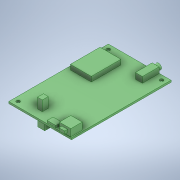
# Autodesk Inventor part: ECG PCB
Saved by Autodesk Inventor 2020 (Build 240168000, 168)
## iProperties
Created: 2021-04-18
Part Number: ECG PCB
Material: Generic
Document SubType Name: Modeling
Designer: Karl
Density: 1 g/cm^3
Appearance: Smooth - Dark Forest Green
Author: Karl
Autodesk Inventor part; units mm, degrees
ref_plane "YZ Plane" through (0, 0, 0) normal (1, 0, 0) x (0, 1, 0)
ref_plane "XZ Plane" through (0, 0, 0) normal (0, 1, 0) x (-1, 0, 0)
ref_plane "XY Plane" through (0, 0, 0) normal (0, 0, 1) x (1, 0, 0)
sketch "Sketch1" plane through (0, 0, 0) normal (0, 1, 0) x (-1, 0, 0)
  line L0 (-26.9875, 42.8625) -> (26.9875, 42.8625)
  line L1 (26.9875, 42.8625) -> (26.9875, -42.8625)
  line L2 (26.9875, -42.8625) -> (-26.9875, -42.8625)
  line L3 (-26.9875, -42.8625) -> (-26.9875, 42.8625)
  line L4 (-26.9875, 42.8625) -> (26.9875, -42.8625) construction
  line L5 (26.9875, 42.8625) -> (-26.9875, -42.8625) construction
  point P0 (0, 0)
  dimension "d0" = 53.975
  dimension "d1" = 85.725
  constraints: 12 end point, 2 midpoint, 2 parallel, 1 horizontal, 1 perpendicular
  measures "d0" distance of L1.end L2.end
  measures "d1" distance of L0.end L1.end
extrude "Extrusion1" add sketch "Sketch1" along normal blind 1.57
sketch "Sketch2" plane through (0, 1.57, 0) normal (0, 1, 0) x (1, 0, 0)
  line L0 (-26.9875, -42.8625) -> (26.9875, -42.8625) projected
  line L1 (-26.9875, 42.8625) -> (-26.9875, -42.8625) projected
  line L2 (26.9875, 42.8625) -> (-26.9875, 42.8625) projected
  line L3 (26.9875, -42.8625) -> (26.9875, 42.8625) projected
  point P0 (0, 0)
  point P1 (-22.9235, -38.7985)
  point P2 (-22.9235, 38.7985)
  point P3 (22.9235, 38.7985)
  dimension "d4" = 4.064
  dimension "d5" = 4.064
  dimension "d6" = 4.064
  dimension "d7" = 4.064
  dimension "d8" = 4.064
  dimension "d9" = 4.064
  measures "d4" distance from line of L0 point (-22.923, -38.798)
  measures "d5" distance from line of L1 point (-22.923, -38.798)
  measures "d6" distance from line of L1 point (-22.923, 38.798)
  measures "d7" distance from line of point (-22.923, 38.798) L2
  measures "d8" distance from line of L2 point (22.923, 38.798)
  measures "d9" distance from line of L3 point (22.923, 38.798)
hole "Hole1" at (-22.9235, 1.57, 38.7985) at (-22.9235, 1.57, -38.7985) at (22.9235, 1.57, -38.7985) direction (0, -1, 0) diameter 3 depth 2.54
sketch "Sketch3" plane through (0, 1.57, 0) normal (0, 1, 0) x (1, 0, 0)
  line L0 (26.9875, -42.8625) -> (26.9875, 42.8625) projected
  line L1 (26.9875, 42.8625) -> (-26.9875, 42.8625) projected
  line L2 (16.9065, 28.2465) -> (10.9065, 28.2465)
  line L3 (10.9065, 28.2465) -> (10.9065, 42.7465)
  line L4 (10.9065, 42.7465) -> (16.9065, 42.7465)
  line L5 (16.9065, 42.7465) -> (16.9065, 28.2465)
  line L6 (16.9065, 28.2465) -> (10.9065, 42.7465) construction
  line L7 (10.9065, 28.2465) -> (16.9065, 42.7465) construction
  point P0 (0, 0)
  point P1 (13.9065, 35.4965)
  dimension "d17" = 13.081
  dimension "d18" = 7.366
  dimension "d19" = 14.5
  dimension "d20" = 6
  constraints: 12 end point, 2 midpoint, 2 parallel, 1 horizontal, 1 perpendicular
  measures "d17" distance from line of L0 point (13.906, 35.496)
  measures "d18" distance from line of L1 point (13.906, 35.496)
  measures "d19" distance of L2.end L3.end
  measures "d20" distance of L2.start L2.end
extrude "Extrusion2" add sketch "Sketch3" along normal blind 5
sketch "Sketch4" plane through (16.9065, 1.57, -42.7465) normal (0, 0, -1) x (-1, 0, 0)
  line L0 (6, 0) -> (6, 5) projected
  circle A0 centre (3, 2.5) radius 2.5
  point P0 (16.9065, -1.57)
  dimension "d23" = 5
  constraints: 1 centre point
  measures "d23" diameter of A0
extrude "Extrusion3" add sketch "Sketch4" along normal blind 2.5
sketch "Sketch5" plane through (0, 1.57, 0) normal (0, 1, 0) x (1, 0, 0)
  line L0 (-26.9875, -42.8625) -> (26.9875, -42.8625) projected
  line L1 (26.9875, -42.8625) -> (26.9875, 42.8625) projected
  line L2 (-4.9284, -30.8693) -> (-9.1184, -30.8693)
  line L3 (-9.1184, -30.8693) -> (-9.1184, -36.0693)
  line L4 (-9.1184, -36.0693) -> (-4.9284, -36.0693)
  line L5 (-4.9284, -36.0693) -> (-4.9284, -30.8693)
  line L6 (-4.9284, -30.8693) -> (-9.1184, -36.0693) construction
  line L7 (-9.1184, -30.8693) -> (-4.9284, -36.0693) construction
  point P0 (0, 0)
  point P1 (-7.3025, -33.9725)
  point P2 (-7.0234, -33.4693)
  dimension "d26" = 8.89
  dimension "d27" = 34.29
  dimension "d28" = 5.2
  dimension "d29" = 4.19
  constraints: 12 end point, 2 midpoint, 2 parallel, 1 horizontal, 1 perpendicular
  measures "d26" distance from line of point (-7.303, -33.973) L0
  measures "d27" distance from line of L1 point (-7.303, -33.973)
  measures "d28" distance of L2.end L3.end
  measures "d29" distance of L3.end L4.end
extrude "Extrusion4" add sketch "Sketch5" along normal blind 8.77
sketch "Sketch6" plane through (0, 1.57, 0) normal (0, 1, 0) x (1, 0, 0)
  line L0 (-6.0004, 7.1846) -> (-24.0004, 7.1846)
  line L1 (-24.0004, 7.1846) -> (-24.0004, 32.6846)
  line L2 (-24.0004, 32.6846) -> (-6.0004, 32.6846)
  line L3 (-6.0004, 32.6846) -> (-6.0004, 7.1846)
  line L4 (-6.0004, 7.1846) -> (-24.0004, 32.6846) construction
  line L5 (-24.0004, 7.1846) -> (-6.0004, 32.6846) construction
  point P0 (0, 0)
  point P1 (-15.0004, 19.9346)
  dimension "d34" = 25.5
  dimension "d35" = 18
  constraints: 12 end point, 2 midpoint, 2 parallel, 1 horizontal, 1 perpendicular
  measures "d34" distance of L0.end L1.end
  measures "d35" distance of L0.start L0.end
extrude "Extrusion5" add sketch "Sketch6" along normal blind 4.2
sketch "Sketch7" plane through (0, 0, 0) normal (0, -1, 0) x (1, 0, 0)
  line L0 (2.7595, 37.1835) -> (-3.1405, 37.1835)
  line L1 (-3.1405, 37.1835) -> (-3.1405, 41.6835)
  line L2 (-3.1405, 41.6835) -> (2.7595, 41.6835)
  line L3 (2.7595, 41.6835) -> (2.7595, 37.1835)
  line L4 (2.7595, 37.1835) -> (-3.1405, 41.6835) construction
  line L5 (-3.1405, 37.1835) -> (2.7595, 41.6835) construction
  line L6 (-26.9875, 42.8625) -> (26.9875, 42.8625) projected
  line L7 (-26.9875, -42.8625) -> (-26.9875, 42.8625) projected
  line L8 (26.9875, 42.8625) -> (26.9875, -42.8625) projected
  point P0 (0, 0)
  point P1 (-0.1905, 39.4335)
  dimension "d36" = 4.5
  dimension "d37" = 5.9
  dimension "d38" = 3.429
  dimension "d40" = 27.178
  constraints: 12 end point, 2 midpoint, 2 parallel, 1 horizontal, 1 perpendicular
  measures "d36" distance of L2.end L0.start
  measures "d37" distance of L0.start L0.end
  measures "d38" distance from line of L6 point (-0.191, 39.433)
  measures "d40" distance from line of L8 point (-0.191, 39.433)
extrude "Extrusion6" add sketch "Sketch7" along normal blind 6
sketch "Sketch8" plane through (0, 1.57, 0) normal (0, 1, 0) x (1, 0, 0)
  line L0 (26.0985, -42.6085) -> (16.2941, -42.6085)
  line L1 (16.2941, -42.6085) -> (16.2941, -32.7279)
  line L2 (16.2941, -32.7279) -> (26.0985, -32.7279)
  line L3 (26.0985, -32.7279) -> (26.0985, -42.6085)
  line L4 (26.0985, -42.6085) -> (16.2941, -32.7279) construction
  line L5 (16.2941, -42.6085) -> (26.0985, -32.7279) construction
  line L6 (26.9875, -42.8625) -> (26.9875, 42.8625) projected
  line L7 (-26.9875, -42.8625) -> (26.9875, -42.8625) projected
  point P0 (0, 0)
  point P1 (21.1963, -37.6682)
  dimension "d43" = 9.8044
  dimension "d44" = 9.8806
  dimension "d45" = 0.889
  dimension "d46" = 0.254
  constraints: 12 end point, 2 midpoint, 2 parallel, 1 horizontal, 1 perpendicular
  measures "d43" distance of L1.end L2.end
  measures "d44" distance of L0.end L1.end
  measures "d45" distance between parallel lines of L6 L3
  measures "d46" distance between parallel lines of L0 L7
extrude "Extrusion7" add sketch "Sketch8" along normal blind 6.1722
sketch "Sketch9" plane through (16.2941, 1.57, 42.6085) normal (0, 0, 1) x (1, 0, 0)
  line L0 (0, 0) -> (0, 6.1722) projected
  line L1 (7.0358, 4.2799) -> (2.2606, 4.2799)
  line L2 (2.2606, 4.2799) -> (2.2606, 1.8923)
  line L3 (2.2606, 1.8923) -> (7.0358, 1.8923)
  line L4 (7.0358, 1.8923) -> (7.0358, 4.2799)
  line L5 (7.0358, 4.2799) -> (2.2606, 1.8923) construction
  line L6 (2.2606, 4.2799) -> (7.0358, 1.8923) construction
  line L7 (0, 6.1722) -> (9.8044, 6.1722) projected
  point P0 (-16.2941, -1.57)
  point P1 (4.6482, 3.0861)
  dimension "d52" = 3.0861
  dimension "d53" = 2.2606
  constraints: 12 end point, 2 midpoint, 2 parallel, 1 horizontal, 1 perpendicular
  measures "d52" distance from line of L7 point (4.648, 3.086)
  measures "d53" distance between parallel lines of L0 L2
extrude "Extrusion8" add sketch "Sketch9" along normal blind 2.4892
sketch "Sketch10" plane through (0, 1.57, 0) normal (0, 1, 0) x (1, 0, 0)
  line L0 (26.9875, -42.8625) -> (26.9875, 42.8625) projected
  line L1 (-26.9875, -42.8625) -> (26.9875, -42.8625) projected
  line L2 (13.0175, -42.2275) -> (5.3975, -42.2275)
  line L3 (5.3975, -42.2275) -> (5.3975, -37.1475)
  line L4 (5.3975, -37.1475) -> (13.0175, -37.1475)
  line L5 (13.0175, -37.1475) -> (13.0175, -42.2275)
  line L6 (13.0175, -42.2275) -> (5.3975, -37.1475) construction
  line L7 (5.3975, -42.2275) -> (13.0175, -37.1475) construction
  point P0 (0, 0)
  point P1 (9.2075, -39.6875)
  dimension "d56" = 17.78
  dimension "d57" = 3.175
  dimension "d58" = 7.62
  dimension "d59" = 5.08
  constraints: 12 end point, 2 midpoint, 2 parallel, 1 horizontal, 1 perpendicular
  measures "d56" distance from line of L0 point (9.208, -39.688)
  measures "d57" distance from line of L1 point (9.208, -39.688)
  measures "d58" distance of L3.end L4.end
  measures "d59" distance of L2.end L3.end
extrude "Extrusion9" add sketch "Sketch10" along normal blind 1.8
body "Solid1"
